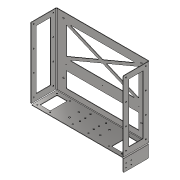
# Autodesk Inventor part: Display_Mount_A
Saved by Autodesk Inventor 2020 (Build 240168000, 168)
## iProperties
Created: 2021-12-05
Part Number: Display_Mount_A
Material: ステンレス鋼
Document SubType Name: Sheet Metal
Designer: ken113
Density: 8 g/cm^3
Sheet Metal Rule: Default_mm
Appearance: 半つや出し
Flat Pattern Width: 55.1048 cm
Flat Pattern Length: 37.0524 cm
Flat Pattern Area: 2041.76 cm^2
Sheet Metal Width: 551.048 mm
Sheet Metal Length: 370.524 mm
Sheet Metal Area: 204176.371 mm^2
Mass: 1808.32 g
Surface Area: 2392.5 cm^2
Volume: 226.04 cm^3
Author: ken113
Autodesk Inventor part; units mm, degrees
ref_plane "YZ Plane" through (0, 0, 0) normal (1, 0, 0) x (0, 1, 0)
ref_plane "XZ Plane" through (0, 0, 0) normal (0, 1, 0) x (-1, 0, 0)
ref_plane "XY Plane" through (0, 0, 0) normal (0, 0, 1) x (1, 0, 0)
sketch "スケッチ1" plane through (0, 0, 0) normal (0, 0, 1) x (1, 0, 0)
  line L0 (175, -135) -> (-175, -135)
  line L1 (-175, -135) -> (-175, 135)
  line L2 (-175, 135) -> (175, 135)
  line L3 (175, 135) -> (175, -135)
  line L4 (175, -135) -> (-175, 135) construction
  line L5 (-175, -135) -> (175, 135) construction
  point P0 (0, 0)
  dimension "d0" = 270
  dimension "d1" = 350
  measures "d0" distance of L0.end L1.end
  measures "d1" distance of L1.end L2.end
extrude "プレート1" add sketch "スケッチ1" along normal blind 2
sketch "スケッチ2" plane through (175, -137, 4) normal (0, -1, 0) x (1, 0, 0)
  line L0 (-350, 0) -> (0, 0)
  line L1 (0, 0) -> (0, 96)
  line L2 (0, 96) -> (-350, 96)
  line L3 (-350, 96) -> (-350, 0)
  constraints: 6 end point, 1 horizontal, 1 perpendicular, 1 vertical
edge flange "フランジ1" height 100 angle 90 thickness 2 bend radius 2 thickness toward (0, -1, 0) relief straight relief width 2 relief depth 1 edges at (0, -135, 2) wall of the first edge with corners at (-175, -137, 4) (175, -137, 4) (175, -137, 100) (-175, -137, 100)
bend "曲げ1"
corner "コーナー1"
sketch "スケッチ3" plane through (0, 0, 2) normal (0, 0, 1) x (1, 0, 0)
  line L0 (150, -85) -> (-150, -85)
  line L1 (-150, -85) -> (-150, 115)
  line L2 (-150, 115) -> (150, 115)
  line L3 (150, 115) -> (150, -85)
  line L4 (150, -85) -> (-150, 115) construction
  line L5 (-150, -85) -> (150, 115) construction
  line L6 (175, -135) -> (-175, -135) projected
  point P0 (0, 0)
  point P1 (0, 15)
  dimension "d13" = 300
  dimension "d14" = 200
  dimension "d15" = 50
  constraints: 12 end point, 2 midpoint, 2 parallel, 1 horizontal, 1 perpendicular
  measures "d13" distance of L0.start L0.end
  measures "d14" distance of L0.end L1.end
  measures "d15" distance between parallel lines of L0 L6
hole "穴1" at (-150, 115, 2) at (-150, -85, 2) at (150, -85, 2) at (150, 115, 2) direction (0, 0, -1) diameter 6.2 depth 2 tip angle 118
sketch "スケッチ4" plane through (0, 0, 2) normal (0, 0, 1) x (1, 0, 0)
  line L0 (140, -15) -> (-140, -15)
  line L1 (-140, -15) -> (-140, 105)
  line L2 (-140, 105) -> (140, 105)
  line L3 (140, 105) -> (140, -15)
  line L4 (140, -15) -> (-140, 105) construction
  line L5 (-140, -15) -> (140, 105) construction
  circle A0 centre (-150, 115) radius 3.1 projected
  point P0 (0, 0)
  point P1 (0, 45)
  point P2 (0, 45)
  dimension "d23" = 120
  dimension "d24" = 10
  dimension "d155" = 10
  constraints: 12 end point, 3 midpoint, 2 parallel, 1 horizontal, 1 perpendicular, 1 vertical alignment
  measures "d23" distance of L2.end L0.start
  measures "d24" distance from line of L2 A0.centre
  measures "d155" distance from line of L1 A0.centre
extrude "押し出し1" cut sketch "スケッチ4" against normal through all contours L0 L1 L2 L3
fillet "フィレット1" radius 2 4 edges at (140, -15, 1) (140, 105, 1) (-140, 105, 1) (-140, -15, 1)
sketch "スケッチ5" plane through (-175, -137, 100) normal (0, 1, 0) x (1, 0, 0)
  line L0 (350, 96) -> (0, 96) projected
  line L1 (0, 0) -> (0, 96) projected
  line L2 (0, 0) -> (350, 0) projected
  line L3 (350, 0) -> (350, 96) projected
  line L4 (145, 14) -> (205, 14)
  line L5 (205, 14) -> (205, 82)
  line L6 (205, 82) -> (145, 82)
  line L7 (145, 82) -> (145, 14)
  line L8 (145, 14) -> (205, 82) construction
  line L9 (205, 14) -> (145, 82) construction
  line L10 (148.5, 38) -> (201.5, 38)
  line L11 (201.5, 38) -> (201.5, 58)
  line L12 (201.5, 58) -> (148.5, 58)
  line L13 (148.5, 58) -> (148.5, 38)
  line L14 (148.5, 38) -> (201.5, 58) construction
  line L15 (201.5, 38) -> (148.5, 58) construction
  point P0 (175, 100)
  point P1 (175, 48)
  point P2 (175, 0)
  point P3 (175, 48)
  point P4 (0, 48)
  point P5 (175, 48)
  dimension "d29" = 60
  dimension "d30" = 68
  dimension "d31" = 53
  dimension "d32" = 20
  constraints: 24 end point, 8 midpoint, 4 parallel, 2 horizontal, 2 perpendicular, 1 horizontal alignment, 1 vertical alignment
  measures "d29" distance of L6.end L5.end
  measures "d30" distance of L5.end L4.end
  measures "d31" distance of L12.end L11.end
  measures "d32" distance of L11.end L10.end
hole "穴2" at (-30, -137, 18) at (-26.5, -137, 42) at (-26.5, -137, 62) at (26.5, -137, 62) at (26.5, -137, 42) at (30, -137, 18) at (30, -137, 86) at (-30, -137, 86) direction (0, -1, 0) diameter 5.3 depth 2 tip angle 118
sketch "スケッチ6" plane through (177, 135, 4) normal (1, 0, 0) x (0, 1, 0)
  line L0 (-270, 0) -> (0, 0)
  line L1 (0, 0) -> (0, 96)
  line L2 (0, 96) -> (-270, 96)
  line L3 (-270, 96) -> (-270, 0)
  constraints: 6 end point, 1 horizontal, 1 perpendicular, 1 vertical
edge flange "フランジ2" height 100 angle 90 thickness 2 bend radius 2 thickness toward (1, 0, 0) relief straight relief width 2 relief depth 1 corner gap 2 corner form 0 edges at (175, 0, 2) (-175, 0, 2) wall of the first edge with corners at (177, -135, 4) (177, 135, 4) (177, 135, 100) (177, -135, 100)
bend "曲げ2"
corner "コーナー2"
fillet "フィレット2" radius 2 5 edges at (-178, 135, 100) (-178, -135, 100) (-175, -138, 100) (178, -135, 100) (178, 135, 100)
sketch "スケッチ7" plane through (179, -135, 4) normal (1, 0, 0) x (0, 0, -1)
  arc A0 (-96, 268) -> (-94, 270) centre (-94, 268) ccw projected
  line L0 (-96, 2) -> (-96, 268) projected
  arc A1 (-94, 0) -> (-96, 2) centre (-94, 2) ccw projected
  line L1 (0, 0) -> (-94, 0) projected
  line L2 (0, 0) -> (0, 270) projected
  line L3 (-94, 270) -> (0, 270)
  line L4 (-10, 260) -> (-10, 16)
  line L5 (-10, 16) -> (-86, 16)
  line L6 (-86, 16) -> (-86, 260)
  line L7 (-86, 260) -> (-10, 260)
  line L8 (-86, 97.3333) -> (-10, 97.3333)
  line L9 (-10, 97.3333) -> (-10, 178.6667)
  line L10 (-10, 178.6667) -> (-86, 178.6667)
  line L11 (-86, 178.6667) -> (-86, 97.3333)
  point P0 (4, 135)
  dimension "d51" = 10
  dimension "d52" = 244
  dimension "d53" = 81.3333
  dimension "d54" = 81.3333
  dimension "d75" = 10
  dimension "d76" = 16
  dimension "d77" = 10
  constraints: 18 end point, 2 centre point, 2 parallel, 2 perpendicular, 2 point on line, 1 horizontal
  measures "d51" distance between parallel lines of L2 L4
  measures "d52" distance of L5.end L6.end
  measures "d53" distance between parallel lines of L7 L10
  measures "d54" distance between parallel lines of L10 L8
  measures "d75" distance between parallel lines of L6 L0
  measures "d76" distance between parallel lines of L5 L1
  measures "d77" distance between parallel lines of L3 L7
hole "穴3" at (179, 125, 90) at (179, 125, 14) at (179, 43.6667, 14) at (179, 43.6667, 90) at (179, -37.6667, 14) at (179, -37.6667, 90) at (179, -119, 90) at (179, -119, 14) direction (-1, 0, 0) diameter 4.3 depth 2 tip angle 118
mirror "ミラー1" about plane through (0, 0, 0) normal (1, 0, 0) of "穴3"
sketch "スケッチ9" plane through (-175, -139, 4) normal (0, -1, 0) x (1, 0, 0)
  line L0 (2, 96) -> (350, 96) projected
  arc A0 (2, 96) -> (0, 94) centre (2, 94) ccw projected
  line L1 (0, 0) -> (0, 94) projected
  line L2 (0, 0) -> (350, 0) projected
  line L3 (350, 96) -> (350, 0) projected
  circle A1 centre (205, 82) radius 2.65 projected
  circle A2 centre (201.5, 38) radius 2.65 projected
  circle A3 centre (148.5, 58) radius 2.65 projected
  circle A4 centre (145, 14) radius 2.65 projected
  circle A5 centre (148.5, 38) radius 2.65 projected
  circle A6 centre (201.5, 58) radius 2.65 projected
  circle A7 centre (205, 14) radius 2.65 projected
  circle A8 centre (145, 82) radius 2.65 projected
  line L4 (12, 86) -> (62, 86)
  line L5 (62, 86) -> (62, 10)
  line L6 (62, 10) -> (12, 10)
  line L7 (12, 10) -> (12, 86)
  line L8 (288, 86) -> (338, 86)
  line L9 (338, 86) -> (338, 10)
  line L10 (338, 10) -> (288, 10)
  line L11 (288, 10) -> (288, 86)
  point P0 (175, -4)
  dimension "d62" = 12
  dimension "d63" = 10
  dimension "d64" = 10
  dimension "d65" = 12
  dimension "d66" = 50
  dimension "d67" = 50
  constraints: 16 end point, 4 parallel, 2 horizontal, 2 perpendicular, 2 point on line
  measures "d62" distance between parallel lines of L7 L1
  measures "d63" distance between parallel lines of L0 L4
  measures "d64" distance between parallel lines of L6 L2
  measures "d65" distance between parallel lines of L3 L9
  measures "d66" distance of L4.start L4.end
  measures "d67" distance of L8.start L8.end
hole "穴4" at (-163, -139, 14) at (-163, -139, 90) at (-113, -139, 90) at (-113, -139, 14) at (113, -139, 14) at (163, -139, 14) at (163, -139, 90) at (113, -139, 90) direction (0, 1, 0) diameter 4.3 depth 2 tip angle 118
sketch "スケッチ10" plane through (-179, -135, 4) normal (-1, 0, 0) x (0, 0, 1)
  line L0 (20, 250) -> (76, 250)
  line L1 (76, 250) -> (76, 23)
  line L2 (76, 23) -> (20, 23)
  line L3 (20, 23) -> (20, 250)
  line L4 (0, 270) -> (94, 270) projected
  line L5 (96, 268) -> (96, 2) projected
  line L6 (0, 270) -> (0, 0) projected
  line L7 (94, 0) -> (0, 0) projected
  point P0 (-4, 135)
  dimension "d78" = 20
  dimension "d79" = 20
  dimension "d80" = 20
  dimension "d81" = 23
  constraints: 8 end point, 2 parallel, 1 horizontal, 1 perpendicular
  measures "d78" distance between parallel lines of L4 L0
  measures "d79" distance between parallel lines of L5 L1
  measures "d80" distance between parallel lines of L6 L3
  measures "d81" distance between parallel lines of L2 L7
extrude "押し出し2" cut sketch "スケッチ10" against normal through all
fillet "フィレット3" radius 2 8 edges at (-178, -112, 24) (-178, -112, 80) (-178, 115, 80) (-178, 115, 24) (178, 115, 24) (178, 115, 80) (178, -112, 80) (178, -112, 24)
sketch "スケッチ11" plane through (0, 0, 2) normal (0, 0, 1) x (1, 0, 0)
  line L0 (-138, 105) -> (138, 105) projected
  arc A0 (140, 103) -> (138, 105) centre (138, 103) ccw projected
  line L1 (140, 103) -> (140, -13) projected
  arc A1 (138, -15) -> (140, -13) centre (138, -13) ccw projected
  line L2 (138, -15) -> (-138, -15) projected
  arc A2 (-140, -13) -> (-138, -15) centre (-138, -13) ccw projected
  line L3 (-140, -13) -> (-140, 103) projected
  arc A3 (-138, 105) -> (-140, 103) centre (-138, 103) ccw projected
  circle A4 centre (150, -85) radius 3.1 projected
  circle A5 centre (-150, 115) radius 3.1 projected
  circle A6 centre (-150, -85) radius 3.1 projected
  circle A7 centre (150, 115) radius 3.1 projected
  line L4 (-175, -135) -> (-175, 135) projected
  line L5 (175, -135) -> (-175, -135) projected
  line L6 (175, 135) -> (175, -135) projected
  line L7 (-175, 135) -> (175, 135) projected
  point P0 (0, 0)
  point P1 (-140, -35)
  point P2 (0, -35)
  point P3 (140, -35)
  dimension "d87" = 140
  dimension "d92" = 20
  constraints: 1 horizontal, 1 vertical alignment, 2 other
  measures "d87" distance of point (-140, -35) point (0, -35)
  measures "d92" distance from line of point (-140, -35) L2
hole "穴5" at (-140, -35, 2) at (0, -35, 2) at (140, -35, 2) direction (0, 0, -1) diameter 2 end through all
sketch "スケッチ13" plane through (0, 0, 2) normal (0, 0, 1) x (1, 0, 0)
  line L0 (-138, 105) -> (138, 105) projected
  arc A0 (140, 103) -> (138, 105) centre (138, 103) ccw projected
  line L1 (140, 103) -> (140, -13) projected
  arc A1 (138, -15) -> (140, -13) centre (138, -13) ccw projected
  line L2 (138, -15) -> (-138, -15) projected
  arc A2 (-140, -13) -> (-138, -15) centre (-138, -13) ccw projected
  line L3 (-140, -13) -> (-140, 103) projected
  arc A3 (-138, 105) -> (-140, 103) centre (-138, 103) ccw projected
  circle A4 centre (150, -85) radius 3.1 projected
  circle A5 centre (-150, 115) radius 3.1 projected
  circle A6 centre (-150, -85) radius 3.1 projected
  circle A7 centre (150, 115) radius 3.1 projected
  line L4 (-175, -135) -> (-175, 135) projected
  line L5 (175, -135) -> (-175, -135) projected
  line L6 (175, 135) -> (175, -135) projected
  line L7 (-175, 135) -> (175, 135) projected
  line L8 (-140, -55) -> (140, -55)
  line L9 (140, -55) -> (140, -115)
  line L10 (140, -115) -> (-140, -115)
  line L11 (-140, -115) -> (-140, -55)
  point P0 (0, 0)
  dimension "d108" = 20
  dimension "d156" = 40
  constraints: 8 end point, 2 parallel, 2 vertical alignment, 1 horizontal, 1 perpendicular
  measures "d108" distance between parallel lines of L10 L5
  measures "d156" distance between parallel lines of L2 L8
extrude "押し出し3" cut sketch "スケッチ13" against normal blind 10 contours L8 L9 L10 L11
fillet "フィレット4" radius 2 4 edges at (-140, -55, 1) (-140, -115, 1) (140, -115, 1) (140, -55, 1)
sketch "スケッチ14" plane through (-175, -137, 4) normal (0, 1, 0) x (1, 0, 0)
  circle A0 centre (338, -86) radius 2.15 projected
  circle A1 centre (288, -10) radius 2.15 projected
  circle A2 centre (62, -86) radius 2.15 projected
  circle A3 centre (12, -10) radius 2.15 projected
  circle A4 centre (12, -86) radius 2.15 projected
  circle A5 centre (62, -10) radius 2.15 projected
  circle A6 centre (338, -10) radius 2.15 projected
  circle A7 centre (288, -86) radius 2.15 projected
  line L0 (350, -96) -> (350, 0) projected
  line L1 (350, 0) -> (0, 0) projected
  line L2 (0, -94) -> (0, 0) projected
  arc A8 (0, -94) -> (2, -96) centre (2, -94) ccw projected
  line L3 (2, -96) -> (350, -96) projected
  line L4 (148.5, -58) -> (201.5, -58)
  line L5 (201.5, -58) -> (201.5, -38)
  line L6 (201.5, -38) -> (148.5, -38)
  line L7 (148.5, -38) -> (148.5, -58)
  line L8 (234, -66) -> (116, -66)
  line L9 (116, -66) -> (116, -30)
  line L10 (116, -30) -> (234, -30)
  line L11 (234, -30) -> (234, -66)
  line L12 (234, -66) -> (116, -30) construction
  line L13 (116, -66) -> (234, -30) construction
  circle A9 centre (148.5, -58) radius 2.65 projected
  circle A10 centre (148.5, -38) radius 2.65 projected
  point P0 (175, 4)
  point P1 (175, -48)
  point P2 (175, -38)
  point P3 (175, -48)
  point P4 (148.5, -48)
  point P5 (175, -48)
  dimension "d112" = 118
  dimension "d113" = 36
  constraints: 20 end point, 6 midpoint, 4 parallel, 2 coincident, 2 horizontal, 2 perpendicular, 1 horizontal alignment, 1 vertical alignment
  measures "d112" distance of L9.end L10.end
  measures "d113" distance of L8.end L9.end
hole "穴9" at (-59, -137, 34) at (-59, -137, 70) at (59, -137, 70) at (59, -137, 34) direction (0, -1, 0) diameter 6.3 end through all
sketch "スケッチ15" plane through (177, -141, 100) normal (1, 0, 0) x (0, 1, 0)
  line L0 (0, -96) -> (0, 0)
  line L1 (0, 0) -> (-46, 0)
  line L2 (-46, 0) -> (-46, -96)
  line L3 (-46, -96) -> (0, -96)
  constraints: 6 end point, 1 horizontal, 1 perpendicular, 1 vertical
edge flange "フランジ3" height 50 angle 90 thickness 2 bend radius 2 thickness toward (1, 0, 0) relief straight relief width 2 relief depth 1 edges at (175, -139, 52) wall of the first edge with corners at (177, -141, 4) (177, -141, 100) (177, -187, 100) (177, -187, 4)
bend "曲げ3"
corner "コーナー3"
fillet "フィレット5" radius 2 2 edges at (178, -187, 100) (178, -187, 4)
sketch "スケッチ16" plane through (179, -141, 100) normal (1, 0, 0) x (0, 0, -1)
  line L0 (10, -34) -> (30, -34)
  line L1 (30, -34) -> (30, -19)
  line L2 (30, -19) -> (10, -19)
  line L3 (10, -19) -> (10, -34)
  line L4 (94, -46) -> (2, -46) projected
  line L5 (0, -44) -> (0, 0) projected
  point P0 (100, 141)
  point P1 (10, -26.5)
  dimension "d132" = 15
  dimension "d133" = 19.5
  dimension "d134" = 10
  dimension "d135" = 20
  constraints: 8 end point, 2 parallel, 1 horizontal, 1 midpoint, 1 perpendicular
  measures "d132" distance of L2.end L0.start
  measures "d133" distance from line of point (10, -26.5) L4
  measures "d134" distance between parallel lines of L3 L5
  measures "d135" distance of L0.start L0.end
hole "穴8" at (179, -160, 90) at (179, -175, 90) at (179, -160, 70) at (179, -175, 70) direction (-1, 0, 0) diameter 3.242 depth 11.8 tip angle 118 thread size "M4x0.7" class "6H" standard "ISO Metric profile"
sketch "スケッチ17" plane through (-175, -137, 98) normal (0, 1, 0) x (1, 0, 0)
  circle A0 centre (234, 28) radius 3.15 projected
  circle A1 centre (116, 64) radius 3.15 projected
  circle A2 centre (116, 28) radius 3.15 projected
  circle A3 centre (234, 64) radius 3.15 projected
  circle A4 centre (338, 8) radius 2.15 projected
  circle A5 centre (288, 84) radius 2.15 projected
  circle A6 centre (62, 8) radius 2.15 projected
  circle A7 centre (12, 84) radius 2.15 projected
  circle A8 centre (12, 8) radius 2.15 projected
  circle A9 centre (62, 84) radius 2.15 projected
  circle A10 centre (338, 84) radius 2.15 projected
  circle A11 centre (288, 8) radius 2.15 projected
  arc A12 (0, 0) -> (2, -2) centre (2, 0) ccw projected
  line L0 (2, -2) -> (350, -2) projected
  line L1 (350, -2) -> (350, 94) projected
  line L2 (350, 94) -> (0, 94) projected
  line L3 (0, 0) -> (0, 94) projected
  circle A13 centre (145, 12) radius 2.65 projected
  circle A14 centre (205, 80) radius 2.65 projected
  circle A15 centre (201.5, 36) radius 2.65 projected
  circle A16 centre (148.5, 56) radius 2.65 projected
  circle A17 centre (145, 80) radius 2.65 projected
  circle A18 centre (148.5, 36) radius 2.65 projected
  circle A19 centre (201.5, 56) radius 2.65 projected
  circle A20 centre (205, 12) radius 2.65 projected
  circle A21 centre (12, 84) radius 2.15 projected
  circle A22 centre (62, 8) radius 2.15 projected
  line L4 (12, 84) -> (62, 84)
  line L5 (62, 84) -> (62, 8)
  line L6 (62, 8) -> (12, 8)
  line L7 (12, 8) -> (12, 84)
  circle A23 centre (288, 8) radius 2.15 projected
  circle A24 centre (338, 84) radius 2.15 projected
  line L8 (288, 8) -> (338, 8)
  line L9 (338, 8) -> (338, 84)
  line L10 (338, 84) -> (288, 84)
  line L11 (288, 84) -> (288, 8)
  line L12 (57, 79) -> (17, 79)
  line L13 (17, 79) -> (17, 13)
  line L14 (17, 13) -> (57, 13)
  line L15 (57, 13) -> (57, 79)
  line L16 (293, 13) -> (333, 13)
  line L17 (333, 13) -> (333, 79)
  line L18 (333, 79) -> (293, 79)
  line L19 (293, 79) -> (293, 13)
  point P0 (175, 98)
  dimension "d150" = 5
  dimension "d151" = 5
  constraints: 32 end point, 8 parallel, 4 perpendicular, 2 horizontal, 6 other
  measures "d150" distance between parallel lines of L4 L12
  measures "d151" distance between parallel lines of L11 L19
extrude "押し出し4" cut sketch "スケッチ17" against normal blind 10 contours L15 L14 L13 L12 | L19 L18 L17 L16
fillet "フィレット6" radius 2 8 edges at (-158, -138, 19) (-158, -138, 85) (-118, -138, 85) (-118, -138, 19) (118, -138, 85) (118, -138, 19) (158, -138, 19) (158, -138, 85)
sketch "スケッチ18" plane through (0, 0, 2) normal (0, 0, 1) x (1, 0, 0)
  line L0 (-138, -55) -> (138, -55) projected
  arc A0 (140, -57) -> (138, -55) centre (138, -57) ccw projected
  line L1 (140, -57) -> (140, -113) projected
  arc A1 (138, -115) -> (140, -113) centre (138, -113) ccw projected
  line L2 (138, -115) -> (-138, -115) projected
  arc A2 (-140, -113) -> (-138, -115) centre (-138, -113) ccw projected
  line L3 (-140, -113) -> (-140, -57) projected
  arc A3 (-138, -55) -> (-140, -57) centre (-138, -57) ccw projected
  circle A4 centre (0, -35) radius 1 projected
  circle A5 centre (-140, -35) radius 1 projected
  circle A6 centre (140, -35) radius 1 projected
  line L4 (-140, -13) -> (-140, 103) projected
  arc A7 (-138, 105) -> (-140, 103) centre (-138, 103) ccw projected
  line L5 (-138, 105) -> (138, 105) projected
  arc A8 (140, 103) -> (138, 105) centre (138, 103) ccw projected
  line L6 (140, 103) -> (140, -13) projected
  arc A9 (138, -15) -> (140, -13) centre (138, -13) ccw projected
  line L7 (138, -15) -> (-138, -15) projected
  arc A10 (-140, -13) -> (-138, -15) centre (-138, -13) ccw projected
  circle A11 centre (150, -85) radius 3.1 projected
  circle A12 centre (-150, 115) radius 3.1 projected
  circle A13 centre (-150, -85) radius 3.1 projected
  circle A14 centre (150, 115) radius 3.1 projected
  line L8 (-175, -135) -> (-175, 135) projected
  line L9 (175, -135) -> (-175, -135) projected
  line L10 (175, 135) -> (175, -135) projected
  line L11 (-175, 135) -> (175, 135) projected
  arc A15 (-138, 105) -> (-140, 103) centre (-138, 103) ccw projected
  line L12 (-138, 103) -> (138, -13) construction
  line L13 (-139.9373, 98.3906) -> (136.0627, -17.6094)
  line L14 (139.9373, -8.3906) -> (-136.0627, 107.6094)
  arc A16 (-136.0627, 107.6094) -> (-139.9373, 98.3906) centre (-138, 103) ccw
  arc A17 (136.0627, -17.6094) -> (139.9373, -8.3906) centre (138, -13) ccw
  arc A18 (-140, -13) -> (-138, -15) centre (-138, -13) ccw projected
  line L15 (138, 103) -> (-138, -13) construction
  line L16 (136.0627, 107.6094) -> (-139.9373, -8.3906)
  line L17 (-136.0627, -17.6094) -> (139.9373, 98.3906)
  arc A19 (139.9373, 98.3906) -> (136.0627, 107.6094) centre (138, 103) ccw
  arc A20 (-139.9373, -8.3906) -> (-136.0627, -17.6094) centre (-138, -13) ccw
  point P0 (0, 0)
  point P1 (0, 45)
  point P2 (0, 45)
  point P3 (0, 50.4237)
  point P4 (-129.8541, 105)
  point P5 (-140, 98.4174)
  point P6 (-12.9046, 45)
  point P7 (-140, -8.4174)
  point P8 (-129.8541, -15)
  point P9 (0, 39.5763)
  point P10 (129.8541, -15)
  point P11 (140, -8.4174)
  point P12 (12.9046, 45)
  point P13 (140, 98.4174)
  point P14 (129.8541, 105)
  dimension "d157" = 10
  dimension "d158" = 10
  constraints: 16 end point, 8 point on circle, 8 tangent, 4 centre point, 2 midpoint, 2 parallel
  measures "d157" diameter of A17
  measures "d158" diameter of A20
extrude "押し出し5" add sketch "スケッチ18" against normal up to surface (2 mm away) contours L4 A20 L16 L13 L17 L7 A10 | L4 A7 L5 L14 L16 L13 A16 | L16 L14 L17 L13 | L13 L17 L14 A17 L6 A9 L7 | L16 L5 A8 L6 A19 L17 L14
fillet "フィレット7" radius 2 12 edges at (-129.8541, -15, 1) (-140, -8.4174, 1) (-140, 98.4174, 1) (-129.8541, 105, 1) (-12.9046, 45, 1) (0, 50.4237, 1) (0, 39.5763, 1) (12.9046, 45, 1) (140, 98.4174, 1) (129.8541, 105, 1) (140, -8.4174, 1) (129.8541, -15, 1)
equation "\"d21\" = Thickness"
equation "\"d38\" = Thickness"
equation "\"d53\" = 0.333333 * d52"
equation "\"d54\" = d53"
equation "\"d60\" = Thickness"
equation "\"d73\" = Thickness"
equation "\"d98\" = Thickness"
equation "\"d148\" = Thickness"
equation "\"d2\" = Thickness"
equation "\"d3\" = BendReliefWidth"
equation "\"d4\" = BendReliefDepth"
equation "\"d5\" = MinimumRemnant"
equation "\"d6\" = TransitionRadius"
equation "\"d9\" = BendRadius"
equation "\"d10\" = CornerReliefSize"
equation "\"d11\" = GapSize"
equation "\"d12\" = JacobiRadiusSize"
equation "\"d40\" = BendReliefWidth"
equation "\"d41\" = BendReliefDepth"
equation "\"d42\" = MinimumRemnant"
equation "\"d43\" = TransitionRadius"
equation "\"d46\" = BendRadius"
equation "\"d47\" = CornerReliefSize"
equation "\"d48\" = GapSize"
equation "\"d49\" = JacobiRadiusSize"
equation "\"d121\" = BendReliefWidth"
equation "\"d122\" = BendReliefDepth"
equation "\"d123\" = MinimumRemnant"
equation "\"d124\" = TransitionRadius"
equation "\"d127\" = BendRadius"
equation "\"d128\" = CornerReliefSize"
equation "\"d129\" = GapSize"
equation "\"d130\" = JacobiRadiusSize"
equation "\"BendRadius\" = Thickness"
equation "\"BendReliefWidth\" = Thickness"
equation "\"BendReliefDepth\" = 0.5 * Thickness"
equation "\"CornerReliefSize\" = 4 * Thickness"
equation "\"MinimumRemnant\" = 2 * Thickness"
equation "\"TransitionRadius\" = BendRadius"
equation "\"JacobiRadiusSize\" = BendRadius"
equation "\"GapSize\" = Thickness"
equation "\"Thickness\" = 2"
